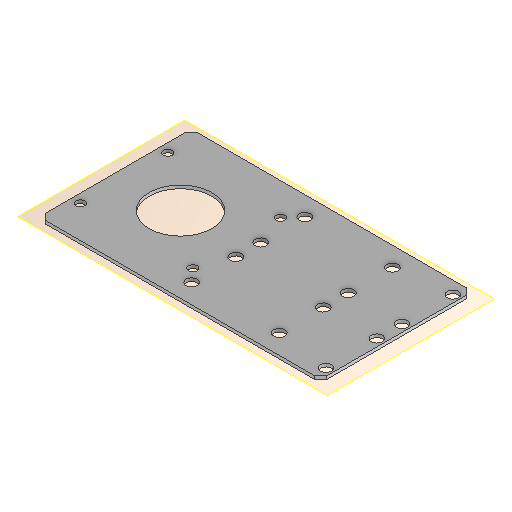
# Autodesk Inventor part: 60_Planktoscope_Sampleholder_spacer
Saved by Autodesk Inventor 2024.1 (Build 281209000, 209)
## iProperties
Created: 2024-07-26
Part Number: 60_Planktoscope_Sampleholder_spacer
Material: Generisch
Document SubType Name: Modeling
Designer: diederichbenedict
Density: 1 g/cm^3
Appearance: Vorgabe
Vendor: openUC2
Mass: 3.90507 g
Surface Area: 83.1638 cm^2
Volume: 3.90507 cm^3
Author: diederichbenedict
Autodesk Inventor part; units mm, degrees
ref_plane "YZ Plane" through (0, 0, 0) normal (1, 0, 0) x (0, 1, 0)
ref_plane "XZ Plane" through (0, 0, 0) normal (0, 1, 0) x (-1, 0, 0)
ref_plane "XY Plane" through (0, 0, 0) normal (0, 0, 1) x (1, 0, 0)
ref_plane "Arbeitsebene1" through (0, 0, 0) normal (0, 0, 1) x (1, 0, 0)
sketch "Skizze1" plane through (0, 0, 0) normal (0, 0, 1) x (1, 0, 0)
  circle A0 centre (-44.65, -14) radius 1.4 projected
  circle A1 centre (-44.65, 14) radius 1.4 projected
  circle A2 centre (-8.65, -14) radius 1.4 projected
  circle A3 centre (-8.65, 14) radius 1.4 projected
  circle A4 centre (23.0201, 18.1) radius 1.8 projected
  circle A5 centre (-4.9799, 18.1) radius 1.8 projected
  circle A6 centre (-4.9799, 4) radius 1.8 projected
  circle A7 centre (-4.9799, -4) radius 1.8 projected
  circle A8 centre (-4.9799, -18.1) radius 1.8 projected
  circle A9 centre (23.0201, -18.1) radius 1.8 projected
  circle A10 centre (23.0201, 4) radius 1.8 projected
  circle A11 centre (23.0201, -4) radius 1.8 projected
  circle A12 centre (40.1702, -4) radius 1.8 projected
  circle A13 centre (40.1702, -20.3) radius 1.8 projected
  circle A14 centre (40.1702, 4) radius 1.8 projected
  circle A15 centre (40.1702, 20.3) radius 1.8 projected
  line L0 (-45.5, -24.3) -> (-47.5, -22.3) projected
  line L1 (40.5, -24.3) -> (-45.5, -24.3) projected
  line L2 (42.5, -22.3) -> (40.5, -24.3) projected
  line L3 (42.5, 22.3) -> (42.5, -22.3) projected
  line L4 (40.5, 24.3) -> (42.5, 22.3) projected
  line L5 (-45.5, 24.3) -> (40.5, 24.3) projected
  line L6 (-47.5, 22.3) -> (-45.5, 24.3) projected
  line L7 (-47.5, -22.3) -> (-47.5, 22.3) projected
  circle A16 centre (-26.65, 0) radius 10 projected
  point P0 (0, 0)
extrude "Extrusion1" add sketch "Skizze1" along normal blind 1
